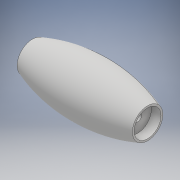
# Autodesk Inventor part: Mecanum_Roller_48mm
Saved by Autodesk Inventor 2018 (Build 220112000, 112)
## iProperties
Created: 2017-08-01
Part Number: Mecanum_Roller_48mm
Material: Generic
Document SubType Name: Modeling
Designer: P136265
Density: 1 g/cm^3
Appearance: Default
Author: P136265
Autodesk Inventor part; units mm, degrees
ref_plane "YZ Plane" through (0, 0, 0) normal (1, 0, 0) x (0, 1, 0)
ref_plane "XZ Plane" through (0, 0, 0) normal (0, 1, 0) x (-1, 0, 0)
sketch "Sketch1" plane through (0, 0, 0) normal (0, 0, 1) x (1, 0, 0)
  circle A0 centre (0, 0) radius 100 construction
  circle A1 centre (0, 0) radius 75 construction
  circle A2 centre (0, 75) radius 24 construction
  circle A3 centre (0, 0) radius 89 construction
  dimension "d8" = 150
  dimension "d7" = 200
  dimension "d9" = 48
  dimension "d10" = 14
  constraints: 3 centre point, 2 coincident, 2 vertical alignment, 2 other
  measures "d7" diameter of A0
  measures "d9" diameter of A2
sketch "Sketch6" plane through (0, 0, 0) normal (0, 0, 1) x (1, 0, 0)
  point P0 (0, 0)
ref_plane "Work Plane3" through (0, 0, 0) normal (0, -0.7071, 0.7071) x (1, 0, 0)
sketch "2d Roller Ellipse" plane through (0, 0, 0) normal (0, -0.7071, 0.7071) x (1, 0, 0)
  ellipse E0 centre (0, 0) end of major axis (100, 0) minor radius 70.7107 construction
  ellipse E1 centre (0, 53.033) end of major axis (24, 53.033) minor radius 16.9706 construction
  ellipse E2 centre (0, 0) end of major axis (100, 0) minor radius 70.7107 construction
  ellipse E3 centre (0, 0) end of major axis (-100, 0) minor radius 70.0036 construction
  line L0 (0, 70.0036) -> (0, 67.0036) construction
  line L1 (0, 67.0036) -> (0, 46.0036) construction
  circle A0 centre (0, 46.0036) radius 21 construction
  ellipse E4 centre (0, 0) end of major axis (-97, 0) minor radius 67.0036 (47.2844, 58.5036) -> (-47.2844, 58.5036) ccw
  line L2 (0, 46.0036) -> (0, 58.5036) construction
  line L3 (0, 58.5036) -> (51.8941, 58.5036) construction
  line L4 (47.2844, 58.5036) -> (47.2844, 46.0036)
  line L5 (47.2844, 46.0036) -> (0, 46.0036)
  line L6 (-47.2844, 58.5036) -> (-47.2844, 46.0036)
  line L7 (-47.2844, 46.0036) -> (0, 46.0036)
  dimension "d53" = 25
  dimension "d61" = 100
  dimension "d63" = 70.7107
  dimension "d77" = 3
  dimension "d78" = 21
  dimension "d79" = 42
  dimension "d80" = 12.5
  dimension "d81" = 12.5
  dimension "d82" = 4.6098
  constraints: 16 end point, 3 coincident, 2 horizontal, 2 point on line, 2 symmetric about line, 2 vertical, 2 vertical alignment, 1 centre point, 1 perpendicular, 11 other
  measures "d77" distance of L0.start L0.end
  measures "d78" distance of L0.end L1.end
  measures "d79" diameter of A0
  measures "d80" distance of L2.start L2.end
  measures "d81" distance of L4.start L4.end
  measures "d82" distance from line of L3.end L4
revolve "Revolution4" add sketch "2d Roller Ellipse" angle 360 about axis through (-47.2844, 32.5294, 32.5294) along (1, 0, 0)
sketch "Sketch11" plane through (47.2844, 32.5294, 32.5294) normal (1, 0, 0) x (0, 0, -1)
  circle A0 centre (0, 0) radius 12.5 projected
  point P0 (32.5294, -32.5294)
  point P1 (-8.8388, 8.8388)
  constraints: 1 other
hole "Hole1" at (47.2844, 32.5294, 32.5294) direction (-1, 0, 0) diameter 6 end through all
sketch "Sketch12" plane through (47.2844, 32.5294, 32.5294) normal (1, 0, 0) x (0, 0, -1)
  circle A0 centre (0, 0) radius 11
  circle A1 centre (0, 0) radius 12.5 projected
  point P0 (32.5294, -32.5294)
  point P1 (-8.8388, 8.8388)
  dimension "d93" = 22
  constraints: 1 centre point, 2 other
  measures "d93" diameter of A0
extrude "Extrusion5" cut sketch "Sketch12" against normal blind 8 contours A0
sketch "Sketch13" plane through (-47.2844, 32.5294, 32.5294) normal (-1, 0, 0) x (0, 0, 1)
  circle A0 centre (0, 0) radius 12.5 projected
  circle A1 centre (0, 0) radius 3 projected
  circle A2 centre (0, 0) radius 11
  point P0 (-32.5294, -32.5294)
  point P1 (8.8388, 8.8388)
  dimension "d96" = 22
  constraints: 1 centre point, 1 coincident, 1 other
  measures "d96" diameter of A2
extrude "Extrusion6" cut sketch "Sketch13" against normal blind 8 contours A2
